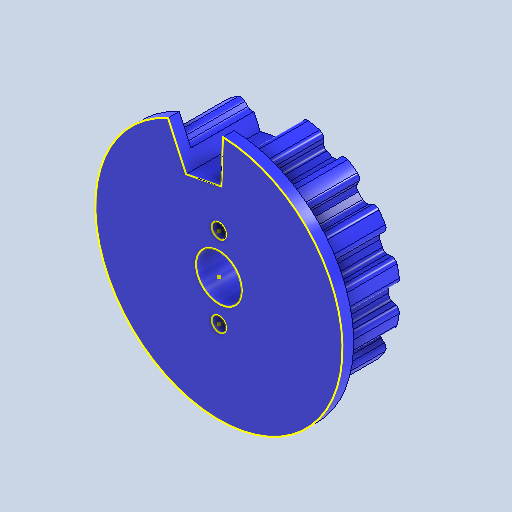
# Autodesk Inventor part: belt_liner_v3_3DP_P-2
Saved by Autodesk Inventor 2025.2 (Build 292293000, 293)
## iProperties
CustomPartVersion: 1
Created: 2024-12-08
Part Number: belt_liner_v3_3DP_P-2
Material: ABS プラスチック
Document SubType Name: Modeling
Designer: haruy
Density: 1.06 g/cm^3
Appearance: 青 - 壁塗料 - 光沢
Author: haruy
Autodesk Inventor part; units mm, degrees
ref_plane "YZ Plane" through (0, 0, 0) normal (1, 0, 0) x (0, 1, 0)
ref_plane "XZ Plane" through (0, 0, 0) normal (0, 1, 0) x (-1, 0, 0)
sketch "プーリ スケッチ" plane through (0, 0, 0) normal (0, 0, 1) x (1, 0, 0)
  circle A0 centre (0, 0) radius 24.2552 construction
  circle A1 centre (0, 0) radius 23.8742
  circle A2 centre (0, 0) radius 21.2072
  line L0 (-2.4489, 23.7483) -> (-1.524, 21.2072)
  line L1 (-1.524, 21.2072) -> (1.524, 21.2072)
  line L2 (1.524, 21.2072) -> (2.4489, 23.7483)
  line L3 (0, 0) -> (0, 23.8742) construction
  point P0 (0, 21.2072)
  dimension "d0" = 48.5104
  dimension "d1" = 0.381
  dimension "d2" = 2.667
  dimension "d3" = 40
  dimension "d4" = 3.048
  constraints: 8 end point, 3 coincident, 3 point on circle, 2 centre point, 1 horizontal, 1 midpoint, 1 point on line, 1 vertical, 1 vertical alignment, 3 other
  measures "d0" diameter of A0
  measures "d1" radial gap between concentric circles of A0 A1
  measures "d3" angle of L2 L0
  measures "d4" distance of L0.end L1.end
extrude "基本ボディ" add sketch "プーリ スケッチ" along normal mid plane 14 contours A2 | A1 L0 L1 L2 | L2 L1 L0 A1
extrude "歯" cut sketch "プーリ スケッチ" along normal through all both and the other way through all contours L2 L1 L0 A1 picked at (0, 22.9759)
fillet "Fillet" radius 1.1938 2 edges at (1.524, 21.2072, 0) (-1.524, 21.2072, 0)
fillet "Fillet" radius 1.1684 4 edges at (-2.4489, 23.7483, 3.5) (-2.4489, 23.7483, -3.5) (2.4489, 23.7483, 3.5) (2.4489, 23.7483, -3.5)
pattern_circular "Teeth" count 16 over 360 about axis through (0, 0, -10) along (0, 0, 1) of "歯", "Fillet"
sketch "スケッチ2" plane through (0, 0, 7) normal (0, 0, 1) x (1, 0, 0)
  circle A0 centre (0, 0) radius 27.5
  dimension "d17" = 55
  constraints: 1 centre point, 1 coincident
  measures "d17" diameter of A0
extrude "押し出し3" add sketch "スケッチ2" along normal blind 2.5
ref_plane "作業平面1" through (0, 0, 0) normal (0, 0, -1) x (-1, 0, 0)
mirror "ミラー1" [suppressed]
sketch "スケッチ3" plane through (0, 0, 9.5) normal (0, 0, 1) x (1, 0, 0)
  circle A0 centre (0, 0) radius 5.1
  circle A1 centre (0, 9) radius 1.6
  circle A2 centre (0, -9) radius 1.6
  dimension "d21" = 10.2
  dimension "d22" = 3.2
  dimension "d23" = 9
  dimension "d26" = 360
  constraints: 3 centre point, 1 coincident, 5 other
  measures "d21" diameter of A0
  measures "d22" diameter of A1
  measures "d23" distance of A1.centre point (0, 0)
extrude "押し出し4" cut sketch "スケッチ3" against normal through all
sketch "スケッチ4" plane through (0, 0, -7) normal (0, 0, -1) x (-1, 0, 0)
  line L0 (-35.8556, 31.439) -> (48.4071, 14.6781)
  arc A0 (5.9069, 23.132) -> (3.395, 23.6316) centre (0, 0) ccw projected
  line L1 (3.395, 23.6316) -> (5.9069, 23.132)
  line L2 (2.199, 23.8695) -> (1.6137, 20.9271)
  line L3 (0, 0) -> (4.6509, 23.3818)
  line L4 (2.6894, 23.772) -> (6.6125, 22.9916)
  line L5 (6.6125, 22.9916) -> (6.2223, 21.03)
  line L6 (6.2223, 21.03) -> (2.2992, 21.8104)
  line L7 (2.2992, 21.8104) -> (2.6894, 23.772)
  line L8 (2.199, 23.8695) -> (7.1029, 22.894)
  line L9 (7.1029, 22.894) -> (9.0538, 32.7019)
  line L10 (9.0538, 32.7019) -> (4.1499, 33.6773)
  line L11 (4.1499, 33.6773) -> (2.199, 23.8695)
  line L12 (-0.1528, 22.2981) -> (8.6743, 20.5423)
  line L13 (8.6743, 20.5423) -> (11.4055, 34.2733)
  line L14 (11.4055, 34.2733) -> (2.5785, 36.0291)
  line L15 (2.5785, 36.0291) -> (-0.1528, 22.2981)
  line L16 (1.118, 26.1237) -> (8.9642, 24.563)
  line L17 (8.9642, 24.563) -> (7.7937, 18.6783)
  line L18 (7.7937, 18.6783) -> (-0.0526, 20.239)
  line L19 (-0.0526, 20.239) -> (1.118, 26.1237)
  line L20 (-0.1528, 22.2981) -> (-0.543, 20.3365)
  line L21 (-0.543, 20.3365) -> (-0.0526, 20.239)
  line L22 (8.6743, 20.5423) -> (8.2841, 18.5807)
  line L23 (8.2841, 18.5807) -> (7.7937, 18.6783)
  line L24 (-11.4055, 34.2733) -> (-8.6743, 20.5423)
  line L25 (-8.6743, 20.5423) -> (-8.2841, 18.5807)
  line L26 (0.0526, 20.239) -> (-7.7937, 18.6783)
  line L27 (-8.2841, 18.5807) -> (-7.7937, 18.6783)
  line L28 (0.543, 20.3365) -> (0.0526, 20.239)
  line L29 (0.1528, 22.2981) -> (0.543, 20.3365)
  line L30 (0.1528, 22.2981) -> (-2.5785, 36.0291)
  line L31 (-23.6532, 27.2997) -> (-15.8752, 15.6591)
  line L32 (-15.8752, 15.6591) -> (-14.764, 13.9962)
  line L33 (-7.6965, 18.7185) -> (-14.3483, 14.2739)
  line L34 (-14.764, 13.9962) -> (-14.3483, 14.2739)
  line L35 (-7.2808, 18.9963) -> (-7.6965, 18.7185)
  line L36 (-8.392, 20.6592) -> (-7.2808, 18.9963)
  line L37 (-8.392, 20.6592) -> (-16.1699, 32.2998)
  line L38 (-32.2998, 16.1699) -> (-20.6592, 8.392)
  line L39 (-20.6592, 8.392) -> (-18.9963, 7.2808)
  line L40 (-14.2739, 14.3483) -> (-18.7185, 7.6965)
  line L41 (-18.9963, 7.2808) -> (-18.7185, 7.6965)
  line L42 (-13.9962, 14.764) -> (-14.2739, 14.3483)
  line L43 (-15.6591, 15.8752) -> (-13.9962, 14.764)
  line L44 (-15.6591, 15.8752) -> (-27.2997, 23.6532)
  line L45 (-36.0291, 2.5785) -> (-22.2981, -0.1528)
  line L46 (-22.2981, -0.1528) -> (-20.3365, -0.543)
  line L47 (-18.6783, 7.7937) -> (-20.239, -0.0526)
  line L48 (-20.3365, -0.543) -> (-20.239, -0.0526)
  line L49 (-18.5807, 8.2841) -> (-18.6783, 7.7937)
  line L50 (-20.5423, 8.6743) -> (-18.5807, 8.2841)
  line L51 (-20.5423, 8.6743) -> (-34.2733, 11.4055)
  line L52 (-34.2733, -11.4055) -> (-20.5423, -8.6743)
  line L53 (-20.5423, -8.6743) -> (-18.5807, -8.2841)
  line L54 (-20.239, 0.0526) -> (-18.6783, -7.7937)
  line L55 (-18.5807, -8.2841) -> (-18.6783, -7.7937)
  line L56 (-20.3365, 0.543) -> (-20.239, 0.0526)
  line L57 (-22.2981, 0.1528) -> (-20.3365, 0.543)
  line L58 (-22.2981, 0.1528) -> (-36.0291, -2.5785)
  line L59 (-27.2997, -23.6532) -> (-15.6591, -15.8752)
  line L60 (-15.6591, -15.8752) -> (-13.9962, -14.764)
  line L61 (-18.7185, -7.6965) -> (-14.2739, -14.3483)
  line L62 (-13.9962, -14.764) -> (-14.2739, -14.3483)
  line L63 (-18.9963, -7.2808) -> (-18.7185, -7.6965)
  line L64 (-20.6592, -8.392) -> (-18.9963, -7.2808)
  line L65 (-20.6592, -8.392) -> (-32.2998, -16.1699)
  line L66 (-16.1699, -32.2998) -> (-8.392, -20.6592)
  line L67 (-8.392, -20.6592) -> (-7.2808, -18.9963)
  line L68 (-14.3483, -14.2739) -> (-7.6965, -18.7185)
  line L69 (-7.2808, -18.9963) -> (-7.6965, -18.7185)
  line L70 (-14.764, -13.9962) -> (-14.3483, -14.2739)
  line L71 (-15.8752, -15.6591) -> (-14.764, -13.9962)
  line L72 (-15.8752, -15.6591) -> (-23.6532, -27.2997)
  line L73 (-2.5785, -36.0291) -> (0.1528, -22.2981)
  line L74 (0.1528, -22.2981) -> (0.543, -20.3365)
  line L75 (-7.7937, -18.6783) -> (0.0526, -20.239)
  line L76 (0.543, -20.3365) -> (0.0526, -20.239)
  line L77 (-8.2841, -18.5807) -> (-7.7937, -18.6783)
  line L78 (-8.6743, -20.5423) -> (-8.2841, -18.5807)
  line L79 (-8.6743, -20.5423) -> (-11.4055, -34.2733)
  line L80 (11.4055, -34.2733) -> (8.6743, -20.5423)
  line L81 (8.6743, -20.5423) -> (8.2841, -18.5807)
  line L82 (-0.0526, -20.239) -> (7.7937, -18.6783)
  line L83 (8.2841, -18.5807) -> (7.7937, -18.6783)
  line L84 (-0.543, -20.3365) -> (-0.0526, -20.239)
  line L85 (-0.1528, -22.2981) -> (-0.543, -20.3365)
  line L86 (-0.1528, -22.2981) -> (2.5785, -36.0291)
  line L87 (23.6532, -27.2997) -> (15.8752, -15.6591)
  line L88 (15.8752, -15.6591) -> (14.764, -13.9962)
  line L89 (7.6965, -18.7185) -> (14.3483, -14.2739)
  line L90 (14.764, -13.9962) -> (14.3483, -14.2739)
  line L91 (7.2808, -18.9963) -> (7.6965, -18.7185)
  line L92 (8.392, -20.6592) -> (7.2808, -18.9963)
  line L93 (8.392, -20.6592) -> (16.1699, -32.2998)
  line L94 (32.2998, -16.1699) -> (20.6592, -8.392)
  line L95 (20.6592, -8.392) -> (18.9963, -7.2808)
  line L96 (14.2739, -14.3483) -> (18.7185, -7.6965)
  line L97 (18.9963, -7.2808) -> (18.7185, -7.6965)
  line L98 (13.9962, -14.764) -> (14.2739, -14.3483)
  line L99 (15.6591, -15.8752) -> (13.9962, -14.764)
  line L100 (15.6591, -15.8752) -> (27.2997, -23.6532)
  line L101 (36.0291, -2.5785) -> (22.2981, 0.1528)
  line L102 (22.2981, 0.1528) -> (20.3365, 0.543)
  line L103 (18.6783, -7.7937) -> (20.239, 0.0526)
  line L104 (20.3365, 0.543) -> (20.239, 0.0526)
  line L105 (18.5807, -8.2841) -> (18.6783, -7.7937)
  line L106 (20.5423, -8.6743) -> (18.5807, -8.2841)
  line L107 (20.5423, -8.6743) -> (34.2733, -11.4055)
  line L108 (34.2733, 11.4055) -> (20.5423, 8.6743)
  line L109 (20.5423, 8.6743) -> (18.5807, 8.2841)
  line L110 (20.239, -0.0526) -> (18.6783, 7.7937)
  line L111 (18.5807, 8.2841) -> (18.6783, 7.7937)
  line L112 (20.3365, -0.543) -> (20.239, -0.0526)
  line L113 (22.2981, -0.1528) -> (20.3365, -0.543)
  line L114 (22.2981, -0.1528) -> (36.0291, 2.5785)
  line L115 (27.2997, 23.6532) -> (15.6591, 15.8752)
  line L116 (15.6591, 15.8752) -> (13.9962, 14.764)
  line L117 (18.7185, 7.6965) -> (14.2739, 14.3483)
  line L118 (13.9962, 14.764) -> (14.2739, 14.3483)
  line L119 (18.9963, 7.2808) -> (18.7185, 7.6965)
  line L120 (20.6592, 8.392) -> (18.9963, 7.2808)
  line L121 (20.6592, 8.392) -> (32.2998, 16.1699)
  line L122 (16.1699, 32.2998) -> (8.392, 20.6592)
  line L123 (8.392, 20.6592) -> (7.2808, 18.9963)
  line L124 (14.3483, 14.2739) -> (7.6965, 18.7185)
  line L125 (7.2808, 18.9963) -> (7.6965, 18.7185)
  line L126 (14.764, 13.9962) -> (14.3483, 14.2739)
  line L127 (15.8752, 15.6591) -> (14.764, 13.9962)
  line L128 (15.8752, 15.6591) -> (23.6532, 27.2997)
  line L129 (13.4918, 31.8191) -> (11.5409, 22.0113)
  line L130 (18.3958, 30.8437) -> (13.4918, 31.8191)
  line L131 (16.4449, 21.0358) -> (18.3958, 30.8437)
  line L132 (11.5409, 22.0113) -> (16.4449, 21.0358)
  line L133 (11.6412, 19.9521) -> (12.0313, 21.9137)
  line L134 (15.5643, 19.1718) -> (11.6412, 19.9521)
  line L135 (15.9545, 21.1334) -> (15.5643, 19.1718)
  line L136 (22.8338, 29.9609) -> (20.8829, 20.153)
  line L137 (27.7377, 28.9854) -> (22.8338, 29.9609)
  line L138 (25.7868, 19.1776) -> (27.7377, 28.9854)
  line L139 (20.8829, 20.153) -> (25.7868, 19.1776)
  line L140 (20.9831, 18.0939) -> (21.3733, 20.0555)
  line L141 (24.9063, 17.3135) -> (20.9831, 18.0939)
  line L142 (25.2965, 19.2751) -> (24.9063, 17.3135)
  circle A1 centre (0, 0) radius 27.5
  line L143 (-0.8791, 27.4859) -> (0.5877, 20.1116)
  line L144 (11.3306, 25.0573) -> (7.1534, 18.8056)
  line L145 (0.3376, 22.2006) -> (8.1839, 20.6398)
  line L146 (8.1839, 20.6398) -> (7.306, 16.2263)
  line L147 (7.306, 16.2263) -> (-0.5403, 17.787)
  line L148 (-0.5403, 17.787) -> (0.3376, 22.2006)
  line L149 (-0.5403, 17.787) -> (-0.8791, 27.4859)
  line L150 (7.306, 16.2263) -> (11.3306, 25.0573)
  point P0 (4.6576, 23.4155)
  point P1 (0.5328, 20.3875)
  point P2 (11.3306, 25.0573)
  point P3 (11.3306, 25.0573)
  point P4 (7.2109, 18.7942)
  point P5 (0.1015, 20.2083)
  point P6 (8.1012, 20.2241)
  point P7 (7.7411, 18.6887)
  point P8 (8.2678, 18.3368)
  point P9 (0.2549, 21.7848)
  point P10 (0, 20.2285)
  point P11 (-0.6213, 20.105)
  point P12 (8.1012, 20.2241)
  point P13 (0.2549, 21.7848)
  dimension "d59" = 55
  dimension "d30" = 0
  dimension "d31" = 2.5
  dimension "d32" = 3
  dimension "d35" = 2
  dimension "d36" = 4
  dimension "d37" = 2
  dimension "d38" = 10
  dimension "d39" = 5
  dimension "d40" = 2.5
  dimension "d41" = 2
  dimension "d42" = 2
  dimension "d45" = 360
  dimension "d49" = 9.525
  dimension "d56" = 4.5
  dimension "d57" = 8
  dimension "d58" = 4
  constraints: 302 end point, 11 parallel, 9 point on line, 6 perpendicular, 3 collinear, 3 symmetric about line, 2 point on circle, 1 coincident, 1 midpoint, 281 other
  measures "d30" distance between parallel lines of L1 L0
  measures "d31" distance from line of L2 point (4.658, 23.415)
  measures "d32" distance from line of L0 L2.end
  measures "d35" distance between parallel lines of L0 L6
  measures "d36" distance between parallel lines of L5 L7
  measures "d37" distance between parallel lines of L3 L7
  measures "d38" distance between parallel lines of L8 L10
  measures "d39" distance between parallel lines of L9 L11
  measures "d40" distance between parallel lines of L3 L11
  measures "d41" distance between parallel lines of L11 L15
  measures "d42" distance between parallel lines of L7 L19
  measures "d49" distance of L10.end L129.start
  measures "d56" distance of L145.end L146.end
  measures "d57" distance between parallel lines of L146 L148
  measures "d58" distance between parallel lines of L3 L148
extrude "押し出し5" cut sketch "スケッチ4" along normal through all both and the other way through all contours L11 L16 L9 L0 A0 | L2 L12 L19 L0 | L0 L7 L12 L2 | L0 L19 L16 L11 | L0 L3 L6 L7 | L19 L12 L29 L30 L15 L0 | L0 L15 A1 L11 L16 L19 | L12 L6 L3 L18 L143 L29 L19 | L11 A1 L9 L16 | A0 L0 | L15 L30 L0 | L0 L30 A1 L15 | L19 L29 L12 | L16 L17 L0 L9 | L9 A1 L13 L0 L17 L16 | L0 L5 L6 L3 | L6 L12 L17 L123 L144 L18 L3 | L30 L15 L20 L21 L148 L26 L149 L0 | L0 L149 L30 | L30 L29 L12 L15 | L29 L19 L21 L20 L12 | L29 L28 L26 L18 L19 | L0 L17 L12 L5 | L18 L124 L146 L147 L3 | L3 L147 L148 L26 L18 | L18 L26 L148 | L143 L18 L26 L28 | A1 L122 L0 L13 | L0 L13 L122 L123 L12 L17 | L144 L125 L124 L18 | L12 L123 L17 | L26 L148 L149 | L0 L122 L13 | L150 L0 L122 | L146 L124 L150 | L124 L125 L123 L17 L18 | L18 L146 L124 | L123 L122 L13 L12 | L12 L22 L23 L17 L123 | L0 L150 L124 L146 L23 L22 L13 L122
sketch "スケッチ5" plane through (0, 0, 9.5) normal (0, 0, 1) x (1, 0, 0)
  arc A0 (-11.3306, 25.0573) -> (0.8791, 27.4859) centre (0, 0) ccw projected
  circle A1 centre (0, -9) radius 1.6 projected
  circle A2 centre (0, 9) radius 1.6 projected
  circle A3 centre (0, 0) radius 5.1 projected
  line L0 (-7.306, 16.2263) -> (-11.3306, 25.0573) projected
  line L1 (0.8791, 27.4859) -> (0.5403, 17.787) projected
  line L2 (0.5403, 17.787) -> (-7.306, 16.2263) projected
sketch "スケッチ6" plane through (0, 0, 9.5) normal (0, 0, 1) x (1, 0, 0)
  line L0 (-7.306, 16.2263) -> (-11.3306, 25.0573) projected
  arc A0 (-11.3306, 25.0573) -> (0.8791, 27.4859) centre (0, 0) ccw projected
  line L1 (0.8791, 27.4859) -> (0.5403, 17.787) projected
  line L2 (0.5403, 17.787) -> (-7.306, 16.2263) projected
  circle A1 centre (0, -9) radius 1.6 projected
  circle A2 centre (0, 9) radius 1.6 projected
  circle A3 centre (0, 0) radius 5.1 projected
equation "\"d1\" = da_a"
equation "\"d2\" = da_hg"
equation "\"d3\" = 2 * da_fi"
equation "\"d4\" = da_bw"
equation "\"d5\" = da_bf"
equation "\"d7\" = da_bf"
equation "\"d9\" = da_rb"
equation "\"d10\" = da_rt"
equation "\"da_pb\" = 9.525"
equation "\"da_fi\" = 20deg"
equation "\"da_hg\" = 2.667"
equation "\"da_bw\" = 3.048"
equation "\"da_rb\" = 1.1938"
equation "\"da_rt\" = 1.1684"
equation "\"da_a\" = 0.381"
equation "\"da_bf\" = 14"
equation "\"da_wf\" = 1.27"
equation "\"da_hf\" = 1.651"
body "Solid1"
